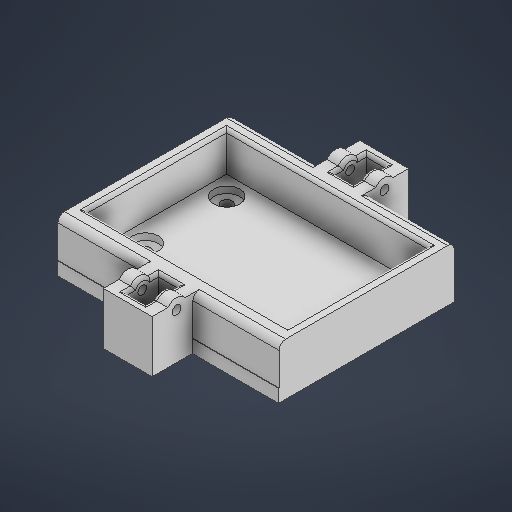
# Autodesk Inventor part: bottomMotorMount
Saved by Autodesk Inventor 2026.2 (Build 302298000, 298)
## iProperties
Created: 2026-09-23
Part Number: bottomMotorMount
Material: Generic
Document SubType Name: Modeling
Designer: Brian Wang
Density: 1 g/cm^3
Appearance: Default
Author: Brian Wang
Autodesk Inventor part; units mm, degrees
ref_plane "YZ Plane" through (0, 0, 0) normal (1, 0, 0) x (0, 1, 0)
ref_plane "XZ Plane" through (0, 0, 0) normal (0, 1, 0) x (-1, 0, 0)
ref_plane "XY Plane" through (0, 0, 0) normal (0, 0, 1) x (1, 0, 0)
sketch "Sketch1" plane through (0, 0, 0) normal (0, 1, 0) x (-1, 0, 0)
  line L0 (7.4046, 11.4154) -> (-60.5954, 11.4154)
  line L1 (-60.5954, 11.4154) -> (-60.5954, -41.5846)
  line L2 (-60.5954, -41.5846) -> (7.4046, -41.5846)
  line L3 (7.4046, -41.5846) -> (7.4046, 11.4154)
  point P0 (0, 0)
  dimension "d0" = 68
  dimension "d1" = 53
  constraints: 8 end point, 2 parallel, 1 horizontal, 1 perpendicular
  measures "d0" distance of L2.end L1.end
  measures "d1" distance of L1.end L0.end
extrude "Extrusion1" add sketch "Sketch1" along normal blind 16
sketch "Sketch2" plane through (0, 16, 0) normal (0, 1, 0) x (1, 0, 0)
  circle A0 centre (1.5954, -2.4154) radius 4
  circle A1 centre (1.5954, 22.5846) radius 4
  circle A2 centre (51.5954, 22.5846) radius 4
  circle A3 centre (51.5954, -2.4154) radius 4
  line L0 (-7.4046, 41.5846) -> (-7.4046, -11.4154) projected
  line L1 (-7.4046, -11.4154) -> (60.5954, -11.4154) projected
  point P0 (0, 0)
  dimension "d4" = 8
  dimension "d5" = 8
  dimension "d6" = 8
  dimension "d7" = 8
  dimension "d8" = 50
  dimension "d9" = 25
  dimension "d10" = 9
  dimension "d11" = 9
  constraints: 4 centre point, 2 horizontal alignment, 2 vertical alignment
  measures "d4" diameter of A0
  measures "d5" diameter of A1
  measures "d6" diameter of A2
  measures "d7" diameter of A3
  measures "d8" distance of A3.centre A0.centre
  measures "d9" distance of A1.centre A0.centre
  measures "d10" distance from line of L0 A0.centre
  measures "d11" distance from line of L1 A0.centre
extrude "Extrusion2" cut sketch "Sketch2" against normal blind 14
sketch "Sketch3" plane through (1.5954, 2, 2.4154) normal (0, 1, 0) x (1, 0, 0)
  circle A0 centre (0, 0) radius 4 projected
  circle A1 centre (0, 0) radius 1.7
  circle A2 centre (0, 25) radius 4 projected
  circle A3 centre (0, 25) radius 1.7
  circle A4 centre (50, 25) radius 4 projected
  circle A5 centre (50, 25) radius 1.7
  circle A6 centre (50, 0) radius 4 projected
  circle A7 centre (50, 0) radius 1.7
  point P0 (-1.5954, 2.4154)
  dimension "d14" = 3.4
  dimension "d15" = 3.4
  dimension "d16" = 3.4
  dimension "d17" = 3.4
  constraints: 4 centre point, 4 coincident
  measures "d14" diameter of A1
  measures "d15" diameter of A3
  measures "d16" diameter of A5
  measures "d17" diameter of A7
extrude "Extrusion3" cut sketch "Sketch3" against normal through all contours A1 | A3 | A5 | A7
sketch "Sketch4" plane through (0, 0, 0) normal (0, -1, 0) x (1, 0, 0)
  line L0 (-7.4046, 11.4154) -> (60.5954, 11.4154) projected
  line L1 (-7.4046, 11.4154) -> (60.5954, 11.4154)
  line L2 (60.5954, 11.4154) -> (60.5954, 32.8654)
  line L3 (60.5954, 32.8654) -> (-7.4046, 32.8654)
  line L4 (-7.4046, 32.8654) -> (-7.4046, 11.4154)
  line L5 (60.5954, -41.5846) -> (-7.4046, -41.5846) projected
  line L6 (-7.4046, -41.5846) -> (60.5954, -41.5846)
  line L7 (60.5954, -41.5846) -> (60.5954, -45.9746)
  line L8 (60.5954, -45.9746) -> (-7.4046, -45.9746)
  line L9 (-7.4046, -45.9746) -> (-7.4046, -41.5846)
  point P0 (0, 0)
  dimension "d20" = 21.45
  dimension "d21" = 4.39
  constraints: 16 end point, 4 parallel, 2 horizontal, 2 perpendicular
  measures "d20" distance of L2.end L1.end
  measures "d21" distance of L6.end L7.end
extrude "Extrusion4" add sketch "Sketch4" against normal blind 16
sketch "Sketch5" plane through (0, 16, 0) normal (0, 1, 0) x (1, 0, 0)
  line L0 (24.0954, 42.9746) -> (29.0954, 42.9746)
  line L1 (29.0954, 42.9746) -> (29.0954, 33.9746)
  line L2 (29.0954, 33.9746) -> (24.0954, 33.9746)
  line L3 (24.0954, 33.9746) -> (24.0954, 42.9746)
  line L4 (24.0954, -20.8654) -> (29.0954, -20.8654)
  line L5 (29.0954, -20.8654) -> (29.0954, -29.8654)
  line L6 (29.0954, -29.8654) -> (24.0954, -29.8654)
  line L7 (24.0954, -29.8654) -> (24.0954, -20.8654)
  line L8 (60.5954, -32.8654) -> (60.5954, 45.9746) projected
  line L9 (60.5954, 45.9746) -> (-7.4046, 45.9746) projected
  line L10 (-7.4046, -32.8654) -> (60.5954, -32.8654) projected
  point P0 (0, 0)
  point P1 (26.5954, 45.9746)
  dimension "d24" = 5
  dimension "d25" = 9
  dimension "d26" = 5
  dimension "d27" = 9
  dimension "d28" = 31.5
  dimension "d29" = 3
  dimension "d30" = 31.5
  dimension "d31" = 3
  constraints: 16 end point, 4 parallel, 2 horizontal, 2 perpendicular, 1 midpoint
  measures "d24" distance of L1.end L2.end
  measures "d25" distance of L0.end L1.end
  measures "d26" distance of L5.end L6.end
  measures "d27" distance of L4.end L5.end
  measures "d28" distance between parallel lines of L8 L1
  measures "d29" distance from line of point (26.595, 45.975) L0
  measures "d30" distance between parallel lines of L8 L5
  measures "d31" distance between parallel lines of L10 L6
extrude "Extrusion5" cut sketch "Sketch5" against normal blind 5
ref_plane "Work Plane1" through (24.0954, 0, 32.8654) normal (1, 0, 0) x (0, 0, -1)
sketch "Sketch6" plane through (24.0954, 0, 32.8654) normal (1, 0, 0) x (0, 0, -1)
  circle A0 centre (7.5, 14.03) radius 4.45
  line L0 (-18.0509, 18.48) -> (105.1295, 18.48)
  line L1 (0, 16) -> (78.84, 16) projected
  circle A1 centre (71.39, 14.03) radius 4.45
  line L2 (75.84, 16) -> (75.84, 11) projected
  circle A2 centre (7.5, 14.03) radius 1.335
  line L3 (7.5, 15.365) -> (7.5, 17.365)
  circle A3 centre (7.5, 14.03) radius 3.335
  circle A4 centre (71.39, 14.03) radius 1.335
  circle A5 centre (71.39, 14.03) radius 3.335
  point P0 (32.8654, 0)
  dimension "d41" = 2.67
  dimension "d35" = 8.9
  dimension "d37" = 2.48
  dimension "d38" = 4.45
  dimension "d39" = 8.9
  dimension "d40" = 4.45
  dimension "d42" = 2
  dimension "d43" = 2.67
  dimension "d44" = 6.67
  constraints: 4 centre point, 4 coincident, 4 end point, 2 vertical alignment, 1 horizontal, 1 perpendicular, 1 tangent, 4 other
  measures "d35" diameter of A0
  measures "d37" distance between parallel lines of L1 L0
  measures "d38" distance from line of L0 A0.centre
  measures "d39" diameter of A1
  measures "d40" distance from line of L0 A1.centre
  measures "d42" distance of L3.start L3.end
  measures "d43" diameter of A4
  measures "d44" diameter of A5
sketch "Sketch7" plane through (24.0954, 0, 32.8654) normal (1, 0, 0) x (0, 0, -1)
  circle A0 centre (7.5, 14.03) radius 4.45
  line L0 (-18.0509, 18.48) -> (105.1295, 18.48)
  circle A1 centre (71.39, 14.03) radius 4.45
  circle A2 centre (7.5, 14.03) radius 1.335
  line L1 (7.5, 15.365) -> (7.5, 17.365)
  circle A3 centre (7.5, 14.03) radius 3.335
  circle A4 centre (71.39, 14.03) radius 1.335
  circle A5 centre (71.39, 14.03) radius 3.335
  line L2 (66.84, 16) -> (75.84, 16) projected
  line L3 (75.84, 16) -> (66.84, 16)
  line L4 (3, 16) -> (12, 16) projected
  line L5 (12, 16) -> (3, 16)
  point P0 (32.8654, 0)
  point P1 (68.699, 16)
  point P2 (74.081, 16)
  point P3 (10.191, 16)
  point P4 (4.809, 16)
  dimension "d50" = 2.67
  dimension "d45" = 8.9
  dimension "d47" = 4.45
  dimension "d48" = 8.9
  dimension "d49" = 4.45
  dimension "d51" = 2
  dimension "d52" = 2.67
  dimension "d53" = 6.67
  constraints: 8 end point, 4 centre point, 4 coincident, 2 horizontal, 1 vertical alignment, 5 other
  measures "d45" diameter of A0
  measures "d47" distance from line of L0 A0.centre
  measures "d48" diameter of A1
  measures "d49" distance from line of L0 A1.centre
  measures "d51" distance of L1.start L1.end
  measures "d52" diameter of A4
  measures "d53" diameter of A5
extrude "Extrusion6" cut sketch "Sketch6" against normal through all contours A2 | A4
extrude "Extrusion7" add sketch "Sketch7" against normal blind 5 contours L4 L1 A3 | A3 L1 L4 | L2 A5 picked at (71.1315, 16.4245)
sketch "Sketch8" plane through (29.0954, 16, -42.9746) normal (-1, 0, 0) x (0, 0, 1)
  circle A0 centre (68.34, -1.97) radius 1.335 projected
  circle A1 centre (68.34, -1.97) radius 1.335
  circle A2 centre (4.45, -1.97) radius 1.335 projected
  circle A3 centre (4.45, -1.97) radius 1.335
  circle A4 centre (4.45, -1.97) radius 3.335
  circle A5 centre (68.34, -1.97) radius 3.335
  point P0 (42.9746, -16)
  constraints: 4 centre point, 4 coincident
extrude "Extrusion8" cut sketch "Sketch8" against normal through all contours A0 | A2
sketch "Sketch9" plane through (29.0954, 16, 20.8654) normal (-1, 0, 0) x (0, 0, 1)
  circle A0 centre (4.5, -1.97) radius 1.335 projected
  circle A1 centre (4.5, -1.97) radius 3.335
  line L0 (9, 0) -> (9, -5) projected
  line L1 (0, 0) -> (0, -5) projected
  line L2 (9, 0) -> (0, 0)
  circle A2 centre (-59.39, -1.97) radius 1.335 projected
  circle A3 centre (-59.39, -1.97) radius 3.335
  line L3 (-63.84, 0) -> (-54.84, 0) projected
  line L4 (-63.6428, 0) -> (-56.3072, 0)
  point P0 (-20.8654, -16)
  point P1 (1.809, 0)
  point P2 (7.191, 0)
  point P3 (-62.081, 0)
  point P4 (-56.699, 0)
  constraints: 4 end point, 2 centre point, 2 coincident, 2 point on line, 1 horizontal
extrude "Extrusion9" add sketch "Sketch9" against normal blind 5 contours L2 A1 | L3 A3 picked at (4.2415, 0.4245) picked at (-59.8259, 0.6151)
sketch "Sketch10" plane through (0, 16, 0) normal (0, 1, 0) x (1, 0, 0)
  line L0 (29.0954, 43.4746) -> (24.0954, 43.4746)
  line L1 (24.0954, 43.4746) -> (24.0954, 33.4746)
  line L2 (24.0954, 33.4746) -> (29.0954, 33.4746)
  line L3 (29.0954, 33.4746) -> (29.0954, 43.4746)
  line L4 (24.0954, 42.9746) -> (29.0954, 42.9746) projected
  line L5 (29.0954, -20.3654) -> (24.0954, -20.3654)
  line L6 (24.0954, -20.3654) -> (24.0954, -30.3654)
  line L7 (24.0954, -30.3654) -> (29.0954, -30.3654)
  line L8 (29.0954, -30.3654) -> (29.0954, -20.3654)
  line L9 (29.0954, -29.8654) -> (24.0954, -29.8654) projected
  point P0 (0, 0)
  dimension "d62" = 10
  dimension "d63" = 0.5
  dimension "d64" = 10
  dimension "d65" = 0.5
  constraints: 16 end point, 4 parallel, 2 horizontal, 2 perpendicular
  measures "d62" distance of L1.end L0.end
  measures "d63" distance between parallel lines of L0 L4
  measures "d64" distance of L6.end L5.end
  measures "d65" distance between parallel lines of L7 L9
extrude "Extrusion10" cut sketch "Sketch10" against normal blind 5
sketch "Sketch11" plane through (-7.4046, 0, -45.9746) normal (-1, 0, 0) x (0, 0, 1)
  line L0 (76.34, 16) -> (76.34, 11) projected
  line L1 (76.34, 16) -> (66.34, 16)
  line L2 (66.34, 16) -> (66.34, 11)
  line L3 (66.34, 11) -> (76.34, 11)
  line L4 (76.34, 11) -> (76.34, 16)
  line L5 (2.5, 16) -> (2.5, 11) projected
  line L6 (2.5, 16) -> (12.5, 16)
  line L7 (12.5, 16) -> (12.5, 11)
  line L8 (12.5, 11) -> (2.5, 11)
  line L9 (2.5, 11) -> (2.5, 16)
  point P0 (45.9746, 0)
  dimension "d68" = 10
  dimension "d69" = 5
  dimension "d70" = 10
  constraints: 16 end point, 4 parallel, 2 horizontal, 2 perpendicular, 1 point on line
  measures "d68" distance of L3.end L2.end
  measures "d69" distance of L2.end L1.end
  measures "d70" distance of L7.end L8.end
extrude "Extrusion11" cut sketch "Sketch11" against normal blind 26.5
sketch "Sketch12" plane through (60.5954, 0, 32.8654) normal (1, 0, 0) x (0, 0, -1)
  line L0 (0, 16) -> (78.84, 16) projected
  line L1 (2.5, 16) -> (12.5, 16)
  line L2 (12.5, 16) -> (12.5, 11)
  line L3 (12.5, 11) -> (2.5, 11)
  line L4 (2.5, 11) -> (2.5, 16)
  line L5 (66.34, 16) -> (76.34, 16)
  line L6 (76.34, 16) -> (76.34, 11)
  line L7 (76.34, 11) -> (66.34, 11)
  line L8 (66.34, 11) -> (66.34, 16)
  point P0 (32.8654, 0)
  point P1 (66.34, 13.5)
  dimension "d73" = 10
  dimension "d74" = 5
  dimension "d75" = 10
  dimension "d76" = 5
  dimension "d78" = 53.84
  constraints: 16 end point, 4 parallel, 2 horizontal, 2 perpendicular, 2 point on line, 1 midpoint, 1 vertical
  measures "d73" distance of L2.end L3.end
  measures "d74" distance of L1.end L2.end
  measures "d75" distance of L6.end L7.end
  measures "d76" distance of L5.end L6.end
  measures "d78" distance from line of point (66.34, 13.5) L2
extrude "Extrusion12" cut sketch "Sketch12" against normal blind 26.5
ref_plane "Work Plane2" through (26.5954, 14.03, 25.3654) normal (1, 0, 0) x (0, 0, -1)
sketch "Sketch13" plane through (26.5954, 14.03, 25.3654) normal (1, 0, 0) x (0, 0, -1)
  line L0 (5, -3.03) -> (-5, -3.03) projected
  line L1 (5, -3.03) -> (-5, -3.03)
  line L2 (-5, -3.03) -> (-5, 11.5918)
  line L3 (-5, 11.5918) -> (5, 11.5918)
  line L4 (5, 11.5918) -> (5, -3.03)
  line L5 (68.84, -3.03) -> (58.84, -3.03) projected
  line L6 (68.84, -3.03) -> (58.84, -3.03)
  line L7 (58.84, -3.03) -> (58.84, 9.9321)
  line L8 (58.84, 9.9321) -> (68.84, 9.9321)
  line L9 (68.84, 9.9321) -> (68.84, -3.03)
  point P0 (25.3654, -14.03)
  constraints: 16 end point, 4 parallel, 2 horizontal, 2 perpendicular
extrude "Extrusion13" cut sketch "Sketch13" along normal mid plane 6.1
sketch "Sketch14" plane through (0, 11, 0) normal (0, 1, 0) x (1, 0, 0)
  line L0 (23.5454, 43.4746) -> (23.5454, 33.4746) projected
  line L1 (23.5454, 43.4746) -> (29.6454, 43.4746)
  line L2 (29.6454, 43.4746) -> (29.6454, 33.4746)
  line L3 (29.6454, 33.4746) -> (23.5454, 33.4746)
  line L4 (23.5454, 33.4746) -> (23.5454, 43.4746)
  line L5 (23.5454, -20.3654) -> (29.6454, -20.3654) projected
  line L6 (23.5454, -30.3654) -> (29.6454, -30.3654) projected
  line L7 (23.5454, -20.3654) -> (29.6454, -20.3654)
  line L8 (29.6454, -20.3654) -> (29.6454, -30.3654)
  line L9 (29.6454, -30.3654) -> (23.5454, -30.3654)
  line L10 (23.5454, -30.3654) -> (23.5454, -20.3654)
  point P0 (0, 0)
  constraints: 16 end point, 4 parallel, 2 horizontal, 2 perpendicular
extrude "Extrusion14" cut sketch "Sketch14" against normal blind 4
fillet "Fillet1" radius 2 4 edges at (47.3454, 16, 20.3654) (5.8454, 16, 20.3654) (47.3454, 16, -33.4746) (5.8454, 16, -33.4746)
fillet "Fillet2" radius 1 8 edges at (23.5454, 16, 21.5199) (23.5454, 17.365, 25.3654) (23.5454, 16, 29.2109) (29.6454, 16, 21.5199) (29.6454, 17.365, 25.3654) (29.6454, 16, 29.2109) (26.5954, 16, 20.3654) (26.5954, 16, 30.3654)
fillet "Fillet3" radius 1 8 edges at (23.5454, 16, -42.3451) (23.5454, 17.365, -38.5246) (23.5454, 16, -34.6541) (26.5954, 16, -43.4746) (29.6454, 16, -42.3451) (29.6454, 17.365, -38.5246) (29.6454, 16, -34.6541) (26.5954, 16, -33.4746)
sketch "Sketch15" plane through (0, 16, 0) normal (0, 1, 0) x (1, 0, 0)
  line L0 (-7.4046, 31.4746) -> (-7.4046, -18.3654) projected
  line L1 (-7.4046, 31.4746) -> (19.0954, 31.4746) projected
  line L2 (60.5954, -18.3654) -> (60.5954, 31.4746) projected
  line L3 (-4.4046, 28.4746) -> (57.5954, 28.4746)
  line L4 (57.5954, 28.4746) -> (57.5954, -14.6478)
  line L5 (57.5954, -14.6478) -> (-4.4046, -14.6478)
  line L6 (-4.4046, -14.6478) -> (-4.4046, 28.4746)
  point P0 (0, 0)
  constraints: 8 end point, 2 parallel, 1 horizontal, 1 perpendicular
extrude "Extrusion15" cut sketch "Sketch15" against normal blind 12
sketch "Sketch16" plane through (60.5954, 11, -33.4746) normal (0, 1, 0) x (1, 0, 0)
  line L0 (-68, 12.5) -> (-68, 10) projected
  line L1 (-41.5, 0) -> (-68, 0) projected
  line L2 (-68, 10) -> (-41.5, 10)
  line L3 (-41.5, 10) -> (-41.5, 0)
  line L4 (-41.5, 0) -> (-68, 0)
  line L5 (-68, 0) -> (-68, 10)
  line L6 (0, 0) -> (0, -2) projected
  line L7 (-26.5, 10) -> (0, 10)
  line L8 (0, 10) -> (0, 0)
  line L9 (0, 0) -> (-26.5, 0)
  line L10 (-26.5, 0) -> (-26.5, 10)
  line L11 (-68, -53.84) -> (-41.5, -53.84) projected
  line L12 (-41.5, -63.84) -> (-68, -63.84) projected
  line L13 (-68, -53.84) -> (-41.5, -53.84)
  line L14 (-41.5, -53.84) -> (-41.5, -63.84)
  line L15 (-41.5, -63.84) -> (-68, -63.84)
  line L16 (-68, -63.84) -> (-68, -53.84)
  line L17 (0, -53.84) -> (-26.5, -53.84) projected
  line L18 (-26.5, -53.84) -> (0, -53.84)
  line L19 (0, -53.84) -> (0, -63.84)
  line L20 (0, -63.84) -> (-26.5, -63.84)
  line L21 (-26.5, -63.84) -> (-26.5, -53.84)
  point P0 (-60.5954, -33.4746)
  constraints: 32 end point, 8 parallel, 4 horizontal, 4 perpendicular, 3 point on line
extrude "Extrusion16" cut sketch "Sketch16" against normal blind 7
fillet "Fillet4" radius 1 4 edges at (-4.4046, 16, -6.9134) (26.5954, 16, -28.4746) (57.5954, 16, -6.9134) (26.5954, 16, 14.6478)
sketch "Sketch17" plane through (0, 16, 0) normal (0, 1, 0) x (1, 0, 0)
  line L0 (-7.4046, 43.4746) -> (19.0954, 43.4746) projected
  line L1 (19.0954, 43.4746) -> (-21.259, 43.4746)
  line L2 (-21.259, 43.4746) -> (-21.259, 53.9968)
  line L3 (-21.259, 53.9968) -> (19.0954, 53.9968)
  line L4 (19.0954, 53.9968) -> (19.0954, 43.4746)
  line L5 (34.0954, 43.4746) -> (60.5954, 43.4746) projected
  line L6 (60.5954, 43.4746) -> (34.0954, 43.4746)
  line L7 (34.0954, 43.4746) -> (34.0954, 51.872)
  line L8 (34.0954, 51.872) -> (60.5954, 51.872)
  line L9 (60.5954, 51.872) -> (60.5954, 43.4746)
  line L10 (60.5954, -30.3654) -> (34.0954, -30.3654) projected
  line L11 (34.0954, -30.3654) -> (75.7941, -30.3654)
  line L12 (75.7941, -30.3654) -> (75.7941, -54.8765)
  line L13 (75.7941, -54.8765) -> (34.0954, -54.8765)
  line L14 (34.0954, -54.8765) -> (34.0954, -30.3654)
  line L15 (19.0954, -30.3654) -> (-7.4046, -30.3654) projected
  line L16 (19.0954, -30.3654) -> (-24.8845, -30.3654)
  line L17 (-24.8845, -30.3654) -> (-24.8845, -57.9495)
  line L18 (-24.8845, -57.9495) -> (19.0954, -57.9495)
  line L19 (19.0954, -57.9495) -> (19.0954, -30.3654)
  point P0 (0, 0)
  constraints: 32 end point, 8 parallel, 4 horizontal, 4 perpendicular
extrude "Extrusion17" cut sketch "Sketch17" against normal blind 12
sketch "Sketch18" plane through (60.5954, 4, -33.4746) normal (0, 1, 0) x (1, 0, 0)
  line L0 (-41.5, -51.84) -> (-41.5, -56.149) projected
  line L1 (-41.5, -53.9945) -> (-74.1891, -53.9945)
  line L2 (-74.1891, -53.9945) -> (-74.1891, -72.5317)
  line L3 (-74.1891, -72.5317) -> (-41.5, -72.5317)
  line L4 (-41.5, -72.5317) -> (-41.5, -53.9945)
  line L5 (-41.5, 0) -> (-68, 0) projected
  line L6 (-41.5, 0) -> (-69.3017, 0)
  line L7 (-69.3017, 0) -> (-69.3017, 14.8194)
  line L8 (-69.3017, 14.8194) -> (-41.5, 14.8194)
  line L9 (-41.5, 14.8194) -> (-41.5, 0)
  line L10 (-26.5, -56.149) -> (-26.5, -51.84) projected
  line L11 (-26.5, -53.9945) -> (6.5925, -53.9945)
  line L12 (6.5925, -53.9945) -> (6.5925, -75.3688)
  line L13 (6.5925, -75.3688) -> (-26.5, -75.3688)
  line L14 (-26.5, -75.3688) -> (-26.5, -53.9945)
  line L15 (-26.5, 0) -> (-26.5, 12.5) projected
  line L16 (-26.5, 0) -> (4.3621, 0)
  line L17 (4.3621, 0) -> (4.3621, 17.3077)
  line L18 (4.3621, 17.3077) -> (-26.5, 17.3077)
  line L19 (-26.5, 17.3077) -> (-26.5, 0)
  point P0 (-60.5954, -33.4746)
  constraints: 32 end point, 8 parallel, 4 horizontal, 4 perpendicular, 2 midpoint
extrude "Extrusion18" cut sketch "Sketch18" against normal blind 12
body "Solid1"
